Autodesk Inventor part; units mm, degrees
(part 2 of 2)
extrude "Выдавливание2" cut sketch "Эскиз3" against normal up to surface (14 mm away) contours A4 A5 A3 A1 picked at (0, 6.5739)
chamfer "Фаска1" distance 0.6 angle 45 2 edges at (0, -7, 9) (0, -7, -5)
chamfer "Фаска2" distance 0.8 angle 45 1 edges at (0, -12.5, 9)
feature "Толщина1" [suppressed]
chamfer "Фаска3" distance 0.5 angle 45 2 edges at (0, -7, -0.5) (0, -7, 4.5)
fillet "Сопряжение1" radius 2 2 edges at (-1.5579, 6.3105, 2) (1.5579, 6.3105, 2)
equation "\"d13\" = d12"
equation "\"Модуль\" = 1"
equation "\"Угол_зацепления\" = 20deg"
equation "\"Зазор_профиля_зуба\" = 0.25"
equation "\"Радиус_закругления_зуба\" = 0.2386"
equation "\"Диаметр_впадин\" = 25.5"
equation "\"Основной_диаметр\" = 26.31139"
equation "\"Средний_диаметр\" = 28"
equation "\"Ширина_грани\" = 5"
equation "\"Коэффициент_смещения\" = 0"
equation "\"Изменение_высоты_головки_зуба\" = 0"
equation "\"Окружной_шаг\" = 3.14159"
equation "\"Общий_сдвиг_инструмента\" = 0"
equation "\"Внутренний\" = 0"
